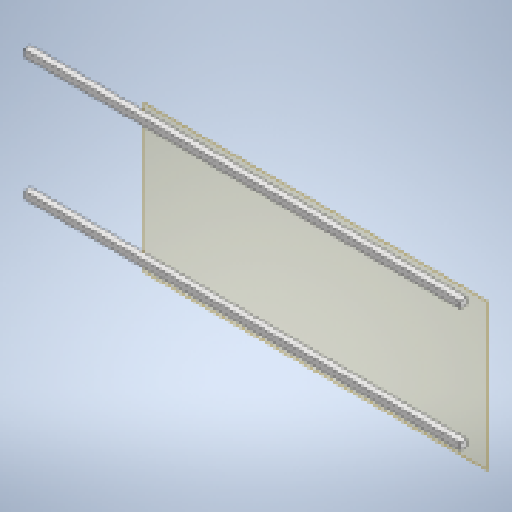
# Autodesk Inventor part: BarrasLargas
Saved by Autodesk Inventor 2024 (Build 280153000, 153)
## iProperties
Created: 2023-07-06
Part Number: BarrasLargas
Material: Genérico
Document SubType Name: Modeling
Designer: sergi
Density: 1 g/cm^3
Appearance: Valor por defecto
Author: sergi
Autodesk Inventor part; units mm, degrees
ref_plane "YZ Plane" through (0, 0, 0) normal (1, 0, 0) x (0, 1, 0)
ref_plane "XZ Plane" through (0, 0, 0) normal (0, 1, 0) x (-1, 0, 0)
ref_plane "Plano de trabajo1" through (0, 0, 0) normal (0, 0, 1) x (1, 0, 0)
sketch "Boceto1" plane through (0, 0, 0) normal (0, 0, 1) x (1, 0, 0)
  line L0 (700, 298.5) -> (700, -298.5) projected
  line L1 (-743, 298.5) -> (700, 298.5) projected
  line L2 (-743, -298.5) -> (-743, 298.5) projected
  line L3 (700, -298.5) -> (-700, -298.5) projected
  line L4 (700, -298.5) -> (675, -298.5) projected
  line L5 (700, 298.5) -> (700, -298.5) projected
  line L6 (675, 298.5) -> (700, 298.5) projected
  line L7 (675, -298.5) -> (675, 298.5) projected
  line L8 (-700, 1251.5) -> (-700, -298.5) projected
  line L9 (-1297, 1251.5) -> (-700, 1251.5) projected
  line L10 (-1297, -358.5) -> (-1297, 1251.5) projected
  line L11 (-700, -298.5) -> (-1297, -298.5) projected
  line L12 (-1281, 1176.5) -> (-1281, -358.5) projected
  line L13 (-1297, 1176.5) -> (-1281, 1176.5) projected
  line L14 (-1297, -358.5) -> (-1297, 1176.5) projected
  line L15 (-1281, -358.5) -> (-1297, -358.5) projected
  line L16 (675, 298.5) -> (-1281, 298.5)
  line L17 (-1281, 298.5) -> (-1281, 268.5)
  line L18 (-1281, 268.5) -> (675, 268.5)
  line L19 (675, 268.5) -> (675, 298.5)
  line L20 (675, -298.5) -> (-1324, -298.5) projected
  line L21 (675, -282.5) -> (675, -298.5) projected
  line L22 (-1324, -282.5) -> (675, -282.5) projected
  line L23 (675, -282.5) -> (-1281, -282.5)
  line L24 (-1281, -282.5) -> (-1281, -252.5)
  line L25 (-1281, -252.5) -> (675, -252.5)
  line L26 (675, -252.5) -> (675, -282.5)
  line L27 (-1324, -298.5) -> (-1324, -282.5) projected
  point P0 (0, 0)
  point P1 (-1281, -282.5)
  point P2 (-1297, -282.5)
  point P3 (-1281, -282.5)
  point P4 (-1281, -282.5)
  point P5 (-1281, -298.5)
  point P6 (-1281, -282.5)
  dimension "d0" = 30
  dimension "d1" = 30
  constraints: 16 end point, 4 parallel, 2 horizontal, 2 perpendicular, 2 point on line, 2 other
  measures "d0" distance of L17.end L16.end
  measures "d1" distance of L23.end L24.end
extrude "Extrusión1" add sketch "Boceto1" along normal blind 30 contours L7 L18 L8 L1 | L3 L8 L22 L7 | L8 L18 L2 L1 | L11 L2 L22 L8 | L22 L8 L25 L7 | L2 L18 L12 L16 | L22 L2 L25 L8 | L11 L12 L22 L2 | L22 L12 L25 L2
